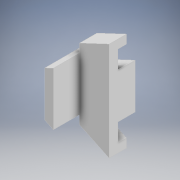
# Autodesk Inventor part: LickPanelLocker
Saved by Autodesk Inventor 2020 (Build 240168000, 168)
## iProperties
Created: 2020-01-17
Part Number: LickPanelLocker
Material: 일반
Document SubType Name: Modeling
Designer: Knowblesse
Density: 1 g/cm^3
Appearance: 기본값
Author: Knowblesse
## iProperties of the stored document _3D 인쇄.ipt
Created: 2020-01-17
Part Number: _3D 인쇄
Material: 일반
Document SubType Name: Modeling
Designer: Knowblesse
Density: 1 g/cm^3
Appearance: 기본값
Author: Knowblesse
Autodesk Inventor part; units mm, degrees
ref_plane "YZ Plane" through (0, 0, 0) normal (1, 0, 0) x (0, 1, 0)
ref_plane "XZ Plane" through (0, 0, 0) normal (0, 1, 0) x (-1, 0, 0)
ref_plane "XY Plane" through (0, 0, 0) normal (0, 0, 1) x (1, 0, 0)
sketch "스케치1" plane through (0, 0, 0) normal (0, 0, 1) x (1, 0, 0)
  line L0 (0, 2.222) -> (0, -2.222)
  line L1 (0, -2.222) -> (22.6058, -12.8981)
  line L2 (22.6058, -12.8981) -> (22.6058, 12.8981)
  line L3 (22.6058, 12.8981) -> (0, 2.222)
  line L4 (0.5, 2.4581) -> (0.5, -2.4581)
  point P0 (0, 0)
  point P1 (0, 0)
  dimension "d0" = 25
  dimension "d1" = 115.28
  dimension "d2" = 115.28
  dimension "d3" = 4.444
  dimension "d4" = 0.5
  constraints: 10 end point, 2 point on line, 2 vertical, 1 coincident, 1 midpoint, 1 parallel
  measures "d0" distance of L2.end L0.start
  measures "d1" angle of L3 L0
  measures "d2" angle of L0 L1
  measures "d3" distance of L0.start L0.end
  measures "d4" distance between parallel lines of L0 L4
extrude "돌출1" add sketch "스케치1" along normal blind 10 contours L3 L2 L1 L4
sketch "스케치2" plane through (0, 0, 10) normal (0, 0, 1) x (1, 0, 0)
  line L0 (0.5, 2.4581) -> (0.5, -2.4581) projected
  line L1 (0.5, -2.4581) -> (22.6058, -12.8981) projected
  line L2 (22.6058, -12.8981) -> (22.6058, 12.8981) projected
  line L3 (22.6058, 12.8981) -> (0.5, 2.4581) projected
  line L4 (0.5, 12.9643) -> (22.6058, 23.4042)
  line L5 (0.5, -12.9643) -> (22.6058, -23.4042)
  line L6 (22.6058, -23.4042) -> (22.6058, -12.8981)
  line L7 (22.6058, -12.8981) -> (22.6058, 12.8981) projected
  line L8 (22.6058, 23.4042) -> (22.6058, 12.8981)
  line L9 (0.5, 12.9643) -> (0.5, 2.4581)
  line L10 (0.5, 2.4581) -> (0.5, -2.4581) projected
  line L11 (0.5, -12.9643) -> (0.5, -2.4581)
  line L12 (22.6058, 12.8981) -> (0.5, 2.4581) projected
  line L13 (0.5, -2.4581) -> (22.6058, -12.8981) projected
  point P0 (0, 0)
  dimension "d23" = 9.5
  dimension "d24" = 9.5
  constraints: 13 end point, 2 collinear, 2 parallel, 2 vertical, 1 point on line
  measures "d23" distance between parallel lines of L5 L1
  measures "d24" distance between parallel lines of L4 L3
extrude "돌출2" add sketch "스케치2" along normal blind 5
sketch "스케치3" plane through (0, 0, 15) normal (0, 0, 1) x (1, 0, 0)
  line L0 (22.6058, -23.4042) -> (22.6058, 23.4042) projected
  line L1 (22.6058, 23.4042) -> (0.5, 12.9643) projected
  line L2 (0.5, 12.9643) -> (0.5, -12.9643) projected
  line L3 (0.5, -12.9643) -> (22.6058, -23.4042) projected
  line L4 (22.6058, 23.4042) -> (0.5, 12.9643) projected
  line L5 (0.5, -12.9643) -> (22.6058, -23.4042) projected
  line L6 (5.5, 15.3256) -> (5.5, -15.3256)
  line L7 (0.5, 12.9643) -> (0.5, -12.9643) projected
  point P0 (0, 0)
  point P1 (5.5, -15.3256)
  dimension "d18" = 5
  constraints: 2 end point, 2 point on line, 1 parallel, 1 vertical
  measures "d18" distance between parallel lines of L6 L2
extrude "돌출3" add sketch "스케치3" along normal blind 15 contours L3 L2 L1 L6
sketch "스케치4" plane through (0, 0, 15) normal (0, 0, 1) x (1, 0, 0)
  line L0 (5.5, 15.3256) -> (5.5, -15.3256) projected
  line L1 (5.5, -15.3256) -> (22.6058, -23.4042) projected
  line L2 (22.6058, -23.4042) -> (22.6058, 23.4042) projected
  line L3 (22.6058, 23.4042) -> (5.5, 15.3256) projected
  line L4 (5.5, 15.3256) -> (5.5, -15.3256) projected
  line L5 (5.5, 15.3256) -> (5.5, 20.3256)
  line L6 (5.5, 20.3256) -> (22.6058, 28.4042)
  line L7 (22.6058, 12.8981) -> (22.6058, 23.4042) projected
  line L8 (22.6058, 28.4042) -> (22.6058, 23.4042)
  line L9 (5.5, -15.3256) -> (5.5, -20.3256)
  line L10 (5.5, -20.3256) -> (22.6058, -28.4042)
  line L11 (22.6058, -28.4042) -> (22.6058, -23.4042)
  line L12 (5.5, -15.3256) -> (22.6058, -23.4042) projected
  point P0 (0, 0)
  dimension "d19" = 5
  dimension "d20" = 5
  constraints: 12 end point, 4 parallel, 2 vertical
  measures "d19" distance of L10.end L1.end
  measures "d20" distance of L6.end L2.end
extrude "돌출4" add sketch "스케치4" against normal blind 10 contours L5 L6 L8 L3 | L1 L11 L10 L9
